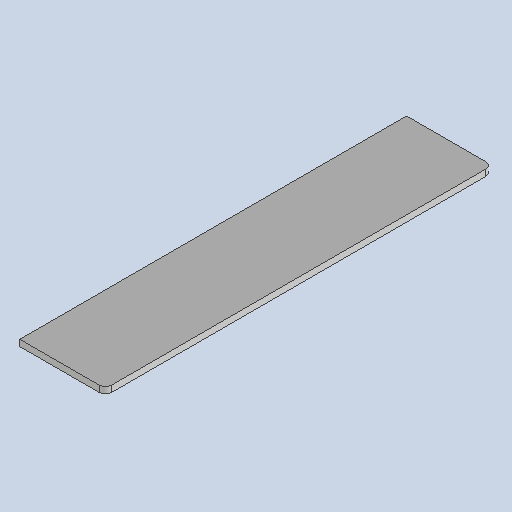
# Autodesk Inventor part: TRM 036 box 1
Saved by Autodesk Inventor 2025 (Build 290162010, 162A)
## iProperties
Created: 2024-08-07
Part Number: TRM 036 box 1
Material: AISI 304
Document SubType Name: Sheet Metal
Designer: user
Stock Number: ТРМ 023 лицо успокоитель
Mass: 52.8588 g
Surface Area: 71.7713 cm^2
Volume: 6.58457 cm^3
Density: 8.02768 g/cm^3
Flat Pattern Width: 12.2 cm
Flat Pattern Length: 2.7 cm
Flat Pattern Area: 32.94 cm^2
Sheet Metal Rule: AISI304 2mm Die16
Sheet Metal Width: 122.000 mm
Sheet Metal Length: 27.000 mm
Sheet Metal Area: 3294.000 mm^2
Appearance: Default
Author: pokla
Autodesk Inventor part; units mm, degrees
ref_plane "YZ Plane" through (0, 0, 0) normal (1, 0, 0) x (0, 1, 0)
ref_plane "XZ Plane" through (0, 0, 0) normal (0, 1, 0) x (-1, 0, 0)
ref_plane "XY Plane" through (0, 0, 0) normal (0, 0, 1) x (1, 0, 0)
sketch "Sketch1" plane through (0, 0, 0) normal (0, 0, 1) x (1, 0, 0)
  line L0 (-13.5, -61) -> (13.5, -61)
  line L1 (13.5, -61) -> (13.5, 61)
  line L2 (13.5, 61) -> (-13.5, 61)
  line L3 (-13.5, 61) -> (-13.5, -61)
  line L4 (-13.5, -61) -> (13.5, 61) construction
  line L5 (13.5, -61) -> (-13.5, 61) construction
  circle A0 centre (-1.5, 51) radius 5.5
  circle A1 centre (-1.5, -51) radius 5.5
  line L6 (-13.5, 0) -> (13.5, 0) construction
  point P0 (0, 0)
  point P1 (0, 0)
  dimension "d0" = 27
  dimension "d1" = 122
  dimension "d12" = 11
  dimension "d13" = 102
  dimension "d15" = 15
  measures "d0" distance of L2.end L1.end
  measures "d1" distance of L1.end L0.end
  measures "d12" diameter of A0
  measures "d13" distance of A1.centre A0.centre
  measures "d15" distance from line of A0.centre L1
extrude "Plate1" add sketch "Sketch1" along normal blind 2 contours L3 L2 L1 L0 | A0 | A1
sketch "Sketch2" plane through (0, 0, 0) normal (0, 0, -1) x (-1, 0, 0)
  line L0 (6.5, 41) -> (206.5, 41) construction
  line L1 (206.5, 41) -> (206.5, 21) construction
  line L2 (206.5, 21) -> (6.5, 21) construction
  line L3 (6.5, 21) -> (6.5, 41) construction
  line L4 (-13.5, 61) -> (13.5, 61) projected
  line L5 (-13.5, -61) -> (-13.5, 61) projected
  point P0 (0, 0)
  point P1 (-48, 100)
  point P2 (13.5, 61)
  point P3 (-50, 98)
  dimension "d6" = 200
  dimension "d9" = 20
  dimension "d10" = 20
  dimension "d11" = 20
  constraints: 4 other
  measures "d6" distance of L0.start L0.end
  measures "d9" distance of L0.end L1.end
  measures "d11" length of L3
mark "Mark1"
fillet "Corner Round1" radius 2 2 edges at (13.5, -61, 1) (13.5, 61, 1)
equation "\"d2\" = Thickness"
equation "\"BendReliefWidth\" = Thickness"
equation "\"BendReliefDepth\" = 0.5 * Thickness"
equation "\"CornerReliefSize\" = 4 * Thickness"
equation "\"MinimumRemnant\" = 2 * Thickness"
equation "\"TransitionRadius\" = BendRadius"
equation "\"JacobiRadiusSize\" = BendRadius"
equation "\"GapSize\" = Thickness"
equation "\"Thickness\" = 2"
equation "\"BendRadius\" = 2.75"
body "Solid1"
